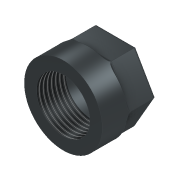
# Autodesk Inventor part: Tapa de Mandril
Saved by Autodesk Inventor 2020.3 (Build 243373000, 373)
## iProperties
Created: 2020-06-07
Part Number: Tapa de Mandril
Material: Iron, Gray
Document SubType Name: Modeling
Designer: Dante
Density: 7.15 g/cm^3
Appearance: Iron Gray
Author: Dante
Autodesk Inventor part; units mm, degrees
ref_plane "YZ Plane" through (0, 0, 0) normal (1, 0, 0) x (0, 1, 0)
ref_plane "XZ Plane" through (0, 0, 0) normal (0, 1, 0) x (-1, 0, 0)
ref_plane "XY Plane" through (0, 0, 0) normal (0, 0, 1) x (1, 0, 0)
sketch "Sketch1" plane through (0, 0, 0) normal (0, 0, 1) x (1, 0, 0)
  circle A0 centre (0, 0) radius 9.5
  circle A1 centre (0, 0) radius 6.5
  line L0 (-9.5, 0) -> (-4.75, 8.227241)
  line L1 (-4.75, 8.227241) -> (4.75, 8.227241)
  line L2 (4.75, 8.227241) -> (9.5, 0)
  line L3 (9.5, 0) -> (4.75, -8.227241)
  line L4 (4.75, -8.227241) -> (-4.75, -8.227241)
  line L5 (-4.75, -8.227241) -> (-9.5, 0)
  circle A2 centre (0, 0) radius 5.5
  circle A3 centre (0, 0) radius 4.25
  dimension "d0" = 19
  dimension "d1" = 13
  dimension "d8" = 11
  dimension "d14" = 8.5
  constraints: 12 end point, 4 coincident, 3 centre point, 16 other
  measures "d1" diameter of A1
  measures "d8" diameter of A2
  measures "d14" diameter of A3
extrude "Extrusion1" add sketch "Sketch1" along normal blind 13 contours L2 A0 | L3 L4 L5 L0 L1 L2 | A0 L3 | L1 A0 | A0 L4 | L0 A0 | A0 L5
extrude "Extrusion2" cut sketch "Sketch1" along normal blind 7 contours L2 A0 | A0 L3 | L1 A0 | A0 L4 | L0 A0 | A0 L5
fillet "Fillet1" radius 1 1 edges at (-7.125, -4.1136, 7)
fillet "Fillet2" radius 1 5 edges at (-7.125, 4.1136, 7) (0, 8.2272, 7) (7.125, 4.1136, 7) (0, -8.2272, 7) (7.125, -4.1136, 7)
extrude "Extrusion3" add sketch "Sketch1" along normal blind 3 contours A1
extrude "Extrusion4" add sketch "Sketch1" along normal blind 3 contours A2
chamfer "Chamfer2" distance 1.5 angle 45 1 edges at (-4.25, 0, 3)
fillet "Fillet3" radius 0.5 6 edges at (-7.125, -4.1136, 0) (0, -8.2272, 0) (-7.125, 4.1136, 0) (0, 8.2272, 0) (7.125, 4.1136, 0) (7.125, -4.1136, 0)
thread "Thread1" size "M14x1" class "6H" standard "ISO Metric profile" length 7
body "Solid1"
